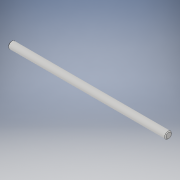
# Autodesk Inventor part: manípulo
Saved by Autodesk Inventor 2017 (Build 210142000, 142)
## iProperties
Created: 2019-10-07
Part Number: manípulo
Material: Generic
Document SubType Name: Modeling
Designer: 20171enpro0154
Density: 1 g/cm^3
Appearance: Default
Author: 20171enpro0154
Autodesk Inventor part; units mm, degrees
ref_plane "YZ Plane" through (0, 0, 0) normal (1, 0, 0) x (0, 1, 0)
ref_plane "XZ Plane" through (0, 0, 0) normal (0, 1, 0) x (-1, 0, 0)
ref_plane "XY Plane" through (0, 0, 0) normal (0, 0, 1) x (1, 0, 0)
sketch "Sketch1" plane through (0, 0, 0) normal (1, 0, 0) x (0, 1, 0)
  circle A0 centre (0, 0) radius 4.7625
  dimension "d0" = 9.525
  constraints: 1 centre point, 1 coincident
  measures "d0" diameter of A0
extrude "Extrusion1" add sketch "Sketch1" along normal blind 220
chamfer "Chamfer1" distance 1 angle 45 2 edges at (220, -4.7625, 0) (0, -4.7625, 0)
body "Solid1"
